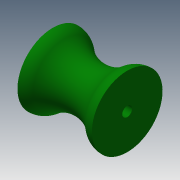
# Autodesk Inventor part: vystuha_hridel_nahore
Saved by Autodesk Inventor 2013 (Build 170138000, 138)
## iProperties
Created: 2013-06-03
Part Number: vystuha_hridel_nahore
Material: Generic
Document SubType Name: Modeling
Designer: idle-rug
Density: 1 g/cm^3
Author: idle-rug
Autodesk Inventor part; units mm, degrees
ref_plane "YZ Plane" through (0, 0, 0) normal (1, 0, 0) x (0, 1, 0)
ref_plane "XZ Plane" through (0, 0, 0) normal (0, 1, 0) x (-1, 0, 0)
ref_plane "XY Plane" through (0, 0, 0) normal (0, 0, 1) x (1, 0, 0)
sketch "Sketch1" plane through (0, 0, 0) normal (0, 1, 0) x (-1, 0, 0)
  line L0 (21.35, -25) -> (26.35, -25)
  line L1 (-21.35, -25) -> (-26.35, -25)
  arc A0 (21.35, -25) -> (-21.35, -25) centre (0, -42.7911) ccw
  line L2 (26.35, 0) -> (-26.35, 0)
  line L3 (-26.35, 0) -> (-26.35, -25)
  line L4 (26.35, 0) -> (26.35, -25)
  point P0 (0, 0)
  dimension "d2" = 5
  dimension "d4" = 5
  constraints: 10 end point, 2 point on circle, 1 centre point, 1 parallel, 1 point on line
  measures "d2" distance of L0.end L0.start
  measures "d4" distance of L1.start L1.end
revolve "Revolution1" add sketch "Sketch1" angle 360 about axis through (-26.35, 0, 0) along (1, 0, 0)
sketch "Sketch2" plane through (-26.35, 0, 0) normal (-1, 0, 0) x (0, 0, 1)
  circle A0 centre (0, 0) radius 25 projected
  circle A1 centre (0, 0) radius 3.5
  dimension "d8" = 7
  constraints: 1 centre point, 1 coincident
  measures "d8" diameter of A1
extrude "Extrusion1" cut sketch "Sketch2" against normal blind 52.7 contours A1
fillet "Fillet1" radius 12 2 edges at (-21.35, 0, 25) (21.35, 0, 25)
body "Solid1"
